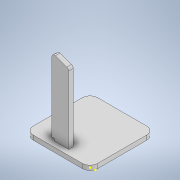
# Autodesk Inventor part: NewBase
Saved by Autodesk Inventor 2020.1 (Build 241239000, 239)
## iProperties
Created: 2020-02-26
Part Number: NewBase
Material: Generic
Document SubType Name: Modeling
Designer: super
Density: 1 g/cm^3
Appearance: Default
Author: super
Autodesk Inventor part; units mm, degrees
ref_plane "YZ Plane" through (0, 0, 0) normal (1, 0, 0) x (0, 1, 0)
ref_plane "XZ Plane" through (0, 0, 0) normal (0, 1, 0) x (-1, 0, 0)
ref_plane "XY Plane" through (0, 0, 0) normal (0, 0, 1) x (1, 0, 0)
sketch "Sketch1" plane through (0, 0, 0) normal (0, 1, 0) x (-1, 0, 0)
  line L0 (0, 0) -> (85, 0)
  line L1 (85, 0) -> (85, -85)
  line L2 (85, -85) -> (0, -85)
  line L3 (0, -85) -> (0, 0)
  dimension "d0" = 85
  dimension "d1" = 85
  constraints: 8 end point, 2 parallel, 1 horizontal, 1 perpendicular
  measures "d0" distance of L1.end L2.end
  measures "d1" distance of L0.end L1.end
extrude "Extrusion1" add sketch "Sketch1" along normal blind 6
fillet "Fillet1" radius 10 4 edges at (-85, 3, 0) (0, 3, 0) (0, 3, -85) (-85, 3, -85)
sketch "Sketch2" plane through (0, 6, 0) normal (0, 1, 0) x (1, 0, 0)
  line L0 (-75, 0) -> (-10, 0) projected
  line L1 (-57, 6.8542) -> (-35, 6.8542)
  line L2 (-35, 6.8542) -> (-35, 11.8542)
  line L3 (-35, 11.8542) -> (-35, 12.8542)
  line L4 (-35, 12.8542) -> (-57, 12.8542)
  line L5 (-57, 12.8542) -> (-57, 6.8542)
  point P0 (0, 0)
  constraints: 10 end point, 3 perpendicular, 1 point on line
extrude "Extrusion2" add sketch "Sketch2" along normal blind 100
sketch "Sketch3" plane through (-57, 6, -6.8542) normal (0, 0, 1) x (1, 0, 0)
  line L0 (22, 100) -> (0, 100) projected
  line L1 (0, 100) -> (22, 100)
  line L2 (22, 100) -> (22, 92.8)
  line L3 (22, 0) -> (22, 100) projected
  line L4 (0, 0) -> (0, 100) projected
  line L5 (0, 100) -> (22, 91.9927)
  line L6 (0, 100) -> (23.4119, 100) construction
  line L7 (22, 91.9927) -> (22, 100)
  point P0 (57, -6)
  dimension "d12" = 7.2
  dimension "d13" = 20
  constraints: 10 end point, 2 point on line, 1 collinear, 1 equal length, 1 horizontal, 1 perpendicular
  measures "d12" distance of L0.start L2.end
  measures "d13" angle of L5 L6
extrude "Extrusion3" cut sketch "Sketch3" against normal blind 10
fillet "Fillet2" radius 3.5 2 edges at (-57, 106, -9.8542) (-35, 97.9927, -9.8542)
sketch "Sketch4" plane through (0, 6, 0) normal (0, 1, 0) x (1, 0, 0)
  point P0 (0, 0)
sketch "Sketch5" plane through (0, 6, 0) normal (0, 1, 0) x (1, 0, 0)
  line L0 (-57, 6.8542) -> (-57, 12.8542) projected
  line L1 (-57, 9.8542) -> (-55.64, 9.8542)
  circle A0 centre (-55.64, 9.8542) radius 1.36
  point P0 (0, 0)
  dimension "d19" = 2.72
  constraints: 2 end point, 1 centre point, 1 coincident, 1 horizontal, 1 midpoint
  measures "d19" diameter of A0
extrude "Extrusion4" add sketch "Sketch5" along normal blind 100
sketch "Sketch6" plane through (-55.64, 106, -9.8542) normal (0, 1, 0) x (1, 0, 0)
  circle A0 centre (0, 0) radius 1.36
  point P0 (55.64, -9.8542)
  constraints: 1 centre point
extrude "Extrusion5" cut sketch "Sketch6" against normal blind 100
sketch "Sketch7" plane through (-57, 6, -6.8542) normal (-1, 0, 0) x (0, 0, 1)
  line L0 (-4.36, 97.771) -> (-4.36, 0) projected
  line L1 (-4.36, 97.771) -> (-1.64, 97.771)
  line L2 (-1.64, 97.771) -> (-1.64, 0) projected
  line L3 (-4.36, 97.771) -> (-4.36, 0)
  line L4 (-4.36, 0) -> (-1.64, 0)
  line L5 (-3.1458, 0) -> (6.8542, 0) projected
  line L6 (-1.64, 0) -> (-1.64, 97.771)
  line L7 (0, 98.5015) -> (0, 95.0015) projected
  point P0 (6.8542, -6)
  point P1 (0, 98.2904)
  constraints: 8 end point, 3 point on line, 1 horizontal, 1 parallel, 1 vertical
extrude "Extrusion6" cut sketch "Sketch7" against normal blind 1.36
sketch "Sketch8" plane through (-57, 6, -6.8542) normal (0, 0, 1) x (1, 0, 0)
  point P0 (57, -6)
sketch "Sketch9" plane through (-57, 6, -6.8542) normal (0, 0, 1) x (1, 0, 0)
  line L0 (0, 0) -> (0, 95.0015) projected
  line L1 (1.36, 0) -> (1.36, 97.771) projected
  line L2 (0, 0) -> (1.36, 0)
  line L3 (1.36, 0) -> (1.36, 3.2)
  line L4 (1.36, 3.2) -> (0, 3.2)
  line L5 (0, 3.2) -> (0, 0)
  line L6 (1.36, 0) -> (0, 0)
  line L7 (47, 0) -> (-18, 0) projected
  point P0 (57, -6)
  dimension "d26" = 3.2
  constraints: 10 end point, 3 perpendicular, 1 collinear, 1 point on line
  measures "d26" distance of L1.start L3.end
extrude "Extrusion7" cut sketch "Sketch9" against normal blind 2
sketch "Sketch10" plane through (-35, 6, -6.8542) normal (0, 0, 1) x (1, 0, 0)
  line L0 (-20.64, 3.2) -> (-22, 3.2) projected
  line L1 (-20.64, 3.2) -> (-19.28, 3.2)
  line L2 (-19.28, 3.2) -> (-19.28, 0)
  line L3 (-19.28, 98.4135) -> (-19.28, 0) projected
  line L4 (25, 0) -> (-40, 0) projected
  line L5 (-20.64, 0) -> (-19.28, 0)
  line L6 (-20.64, 0) -> (-20.64, 97.771) projected
  line L7 (-20.64, 0) -> (-20.64, 3.2)
  point P0 (35, -6)
  dimension "d29" = 1.36
  constraints: 8 end point, 2 collinear, 2 point on line, 1 horizontal
  measures "d29" distance of L0.start L1.end
extrude "Extrusion8" cut sketch "Sketch10" against normal blind 3
body "Solid1"
